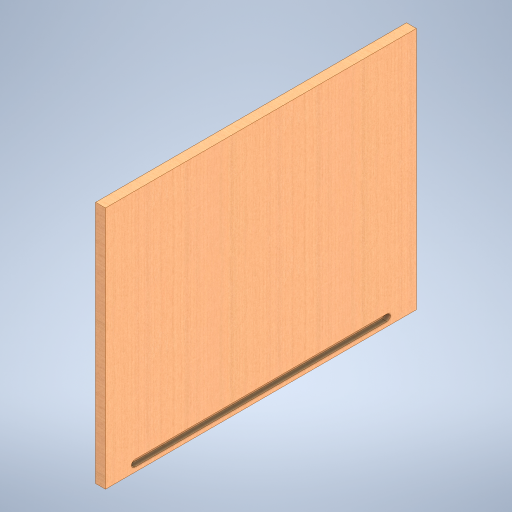
# Autodesk Inventor part: boardTop
Saved by Autodesk Inventor 2024.2 (Build 282272000, 272)
## iProperties
Created: 2024-06-09
Part Number: boardTop
Material: Wood (Cherry)
Document SubType Name: Modeling
Designer: user
Density: 0.63 g/cm^3
Appearance: Cherry - Natural Low Gloss
Author: user
Autodesk Inventor part; units mm, degrees
ref_plane "YZ Plane" through (0, 0, 0) normal (1, 0, 0) x (0, 1, 0)
ref_plane "XZ Plane" through (0, 0, 0) normal (0, 1, 0) x (-1, 0, 0)
ref_plane "XY Plane" through (0, 0, 0) normal (0, 0, 1) x (1, 0, 0)
sketch "Sketch1" plane through (0, 0, 0) normal (1, 0, 0) x (0, 1, 0)
  line L0 (-235, -300) -> (235, -300)
  line L1 (235, -300) -> (235, 300)
  line L2 (235, 300) -> (-235, 300)
  line L3 (-235, 300) -> (-235, -300)
  line L4 (-235, -300) -> (235, 300) construction
  line L5 (235, -300) -> (-235, 300) construction
  point P0 (0, 0)
  dimension "d0" = 470
  dimension "d1" = 600
  constraints: 12 end point, 2 midpoint, 2 parallel, 1 horizontal, 1 perpendicular
  measures "d0" distance of L2.end L1.end
  measures "d1" distance of L1.end L0.end
extrude "Extrusion1" add sketch "Sketch1" along normal blind 19
sketch "Sketch2" plane through (19, 0, 0) normal (1, 0, 0) x (0, 0, -1)
  line L0 (-300, -235) -> (300, -235) projected
  line L1 (243.02, -226.5) -> (-243.02, -226.5)
  line L2 (-250.02, -219.5) -> (-250.02, -220.5)
  line L3 (-243.02, -213.5) -> (243.02, -213.5)
  line L4 (250.02, -220.5) -> (250.02, -219.5)
  line L5 (250.02, -226.5) -> (-250.02, -213.5) construction
  line L6 (-250.02, -226.5) -> (250.02, -213.5) construction
  arc A0 (250.02, -220.5) -> (243.02, -213.5) centre (243.02, -220.5) ccw
  arc A1 (243.02, -226.5) -> (250.02, -219.5) centre (243.02, -219.5) ccw
  arc A2 (-243.02, -213.5) -> (-250.02, -220.5) centre (-243.02, -220.5) ccw
  arc A3 (-250.02, -219.5) -> (-243.02, -226.5) centre (-243.02, -219.5) ccw
  point P0 (0, 0)
  point P1 (0, -220)
  point P2 (250.0021, -220)
  point P3 (-250.0021, -220)
  dimension "d4" = 15
  dimension "d5" = 500.04
  dimension "d6" = 13
  dimension "d7" = 7
  dimension "d8" = 7
  constraints: 12 end point, 8 point on circle, 8 point on line, 8 tangent, 4 centre point, 2 equal radius, 2 midpoint, 2 parallel, 1 horizontal, 1 perpendicular
  measures "d4" distance from line of point (0, -220) L0
  measures "d5" distance of L5.end L6.end
  measures "d6" distance of L6.start L5.end
  measures "d7" radius of A0
  measures "d8" radius of A2
extrude "Extrusion2" cut sketch "Sketch2" against normal blind 10 contours L1 A3 A2 L3 A0 A1
body "Solid1"
